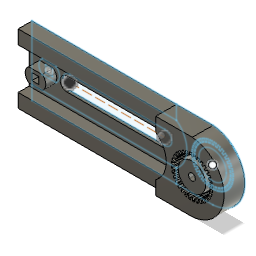
bottom slider mod v1 (Autodesk Fusion 360 design; units mm, degrees)
Autodesk Fusion 360 part; units mm, degrees
sketch "Sketch1" plane through (0, 0, 0) normal (0, 0, 1) x (1, 0, 0)
  line L0 (75, 100) -> (180, 100)
  line L1 (180, 50) -> (75, 50)
  line L2 (75, 50) -> (75, 100)
  line L3 (75, 90) -> (180, 90)
  line L4 (180, 60) -> (75, 60)
  line L5 (85, 77.5) -> (90, 77.5)
  line L6 (90, 77.5) -> (90, 72.5)
  line L7 (90, 72.5) -> (85, 72.5)
  line L8 (85, 72.5) -> (85, 77.5)
  line L9 (82.5, 80) -> (92.5, 80)
  line L10 (92.5, 70) -> (82.5, 70)
  arc A0 (92.5, 70) -> (92.5, 80) centre (88.95, 75) ccw
  arc A1 (82.5, 80) -> (82.5, 70) centre (86.5264, 75) ccw
  line L11 (102.5027, 70) -> (171.6242, 70)
  arc A2 (171.6242, 70) -> (171.6242, 80) centre (171.6242, 75) ccw
  line L12 (171.6242, 80) -> (102.5027, 80)
  arc A3 (102.5027, 80) -> (102.5027, 70) centre (102.5027, 75) ccw
  line L13 (102.5027, 75) -> (171.6242, 75) construction
  arc A4 (180, 60) -> (180, 90) centre (169.0621, 75) ccw
  circle A5 centre (206.3179, 75) radius 10
  circle A6 centre (206.3179, 75) radius 2.5
  line L14 (180, 100) -> (206.5662, 100.0787)
  line L15 (180, 50) -> (206.5662, 50)
  arc A7 (206.5662, 50) -> (206.5662, 100.0787) centre (204.5271, 75.0393) ccw
  line L16 (205.8664, 89.9932) -> (206.0662, 88.0032)
  line L17 (206.0662, 88.0032) -> (207.0662, 88.0032)
  line L18 (207.0662, 88.0032) -> (207.4096, 89.9602)
  line L19 (202.95, 89.617) -> (203.5343, 87.7043)
  line L20 (203.5343, 87.7043) -> (204.5151, 87.8993)
  line L21 (204.5151, 87.8993) -> (204.47, 89.8857)
  line L22 (200.1631, 88.6791) -> (201.1093, 86.9171)
  line L23 (201.1093, 86.9171) -> (202.0332, 87.2998)
  line L24 (202.0332, 87.2998) -> (201.6014, 89.2392)
  line L25 (197.6127, 87.2155) -> (198.8845, 85.6719)
  line L26 (198.8845, 85.6719) -> (199.7159, 86.2275)
  line L27 (199.7159, 86.2275) -> (198.9141, 88.0455)
  line L28 (195.3968, 85.2825) -> (196.9453, 84.0167)
  line L29 (196.9453, 84.0167) -> (197.6524, 84.7238)
  line L30 (197.6524, 84.7238) -> (196.5114, 86.3504)
  line L31 (193.6007, 82.9543) -> (195.3663, 82.0149)
  line L32 (195.3663, 82.0149) -> (195.9219, 82.8464)
  line L33 (195.9219, 82.8464) -> (194.4854, 84.2191)
  line L34 (192.2932, 80.3204) -> (194.2082, 79.7436)
  line L35 (194.2082, 79.7436) -> (194.5909, 80.6675)
  line L36 (194.5909, 80.6675) -> (192.9142, 81.7336)
  line L37 (191.5247, 77.4821) -> (193.5155, 77.2899)
  line L38 (193.5155, 77.2899) -> (193.7106, 78.2707)
  line L39 (193.7106, 78.2707) -> (191.8581, 78.9893)
  line L40 (191.3247, 74.5484) -> (193.3147, 74.7483)
  line L41 (193.3147, 74.7483) -> (193.3147, 75.7483)
  line L42 (193.3147, 75.7483) -> (191.3577, 76.0916)
  line L43 (191.7009, 71.6321) -> (193.6137, 72.2163)
  line L44 (193.6137, 72.2163) -> (193.4186, 73.1971)
  line L45 (193.4186, 73.1971) -> (191.4322, 73.1521)
  line L46 (192.6388, 68.8451) -> (194.4008, 69.7914)
  line L47 (194.4008, 69.7914) -> (194.0182, 70.7152)
  line L48 (194.0182, 70.7152) -> (192.0787, 70.2835)
  line L49 (194.1024, 66.2948) -> (195.646, 67.5665)
  line L50 (195.646, 67.5665) -> (195.0904, 68.398)
  line L51 (195.0904, 68.398) -> (193.2725, 67.5962)
  line L52 (196.0354, 64.0789) -> (197.3012, 65.6274)
  line L53 (197.3012, 65.6274) -> (196.5941, 66.3345)
  line L54 (196.5941, 66.3345) -> (194.9675, 65.1934)
  line L55 (198.3636, 62.2827) -> (199.303, 64.0484)
  line L56 (199.303, 64.0484) -> (198.4715, 64.604)
  line L57 (198.4715, 64.604) -> (197.0988, 63.1675)
  line L58 (200.9975, 60.9753) -> (201.5743, 62.8903)
  line L59 (201.5743, 62.8903) -> (200.6505, 63.273)
  line L60 (200.6505, 63.273) -> (199.5844, 61.5963)
  line L61 (203.8358, 60.2068) -> (204.028, 62.1975)
  line L62 (204.028, 62.1975) -> (203.0472, 62.3926)
  line L63 (203.0472, 62.3926) -> (202.3287, 60.5402)
  line L64 (206.7695, 60.0068) -> (206.5696, 61.9968)
  line L65 (206.5696, 61.9968) -> (205.5696, 61.9968)
  line L66 (205.5696, 61.9968) -> (205.2263, 60.0398)
  line L67 (209.6859, 60.383) -> (209.1016, 62.2957)
  line L68 (209.1016, 62.2957) -> (208.1208, 62.1007)
  line L69 (208.1208, 62.1007) -> (208.1659, 60.1143)
  line L70 (212.4728, 61.3209) -> (211.5266, 63.0829)
  line L71 (211.5266, 63.0829) -> (210.6027, 62.7002)
  line L72 (210.6027, 62.7002) -> (211.0344, 60.7608)
  line L73 (215.0232, 62.7845) -> (213.7514, 64.3281)
  line L74 (213.7514, 64.3281) -> (212.9199, 63.7725)
  line L75 (212.9199, 63.7725) -> (213.7217, 61.9545)
  line L76 (217.239, 64.7175) -> (215.6906, 65.9833)
  line L77 (215.6906, 65.9833) -> (214.9835, 65.2762)
  line L78 (214.9835, 65.2762) -> (216.1245, 63.6496)
  line L79 (219.0352, 67.0457) -> (217.2695, 67.9851)
  line L80 (217.2695, 67.9851) -> (216.714, 67.1536)
  line L81 (216.714, 67.1536) -> (218.1504, 65.7809)
  line L82 (220.3427, 69.6796) -> (218.4277, 70.2564)
  line L83 (218.4277, 70.2564) -> (218.045, 69.3325)
  line L84 (218.045, 69.3325) -> (219.7216, 68.2664)
  line L85 (221.1111, 72.5179) -> (219.1204, 72.7101)
  line L86 (219.1204, 72.7101) -> (218.9253, 71.7293)
  line L87 (218.9253, 71.7293) -> (220.7777, 71.0107)
  line L88 (221.3111, 75.4516) -> (219.3211, 75.2517)
  line L89 (219.3211, 75.2517) -> (219.3211, 74.2517)
  line L90 (219.3211, 74.2517) -> (221.2782, 73.9084)
  line L91 (220.9349, 78.3679) -> (219.0222, 77.7837)
  line L92 (219.0222, 77.7837) -> (219.2173, 76.8029)
  line L93 (219.2173, 76.8029) -> (221.2037, 76.8479)
  line L94 (219.997, 81.1549) -> (218.235, 80.2086)
  line L95 (218.235, 80.2086) -> (218.6177, 79.2848)
  line L96 (218.6177, 79.2848) -> (220.5571, 79.7165)
  line L97 (218.5334, 83.7052) -> (216.9899, 82.4335)
  line L98 (216.9899, 82.4335) -> (217.5454, 81.602)
  line L99 (217.5454, 81.602) -> (219.3634, 82.4038)
  line L100 (216.6004, 85.9211) -> (215.3346, 84.3726)
  line L101 (215.3346, 84.3726) -> (216.0417, 83.6655)
  line L102 (216.0417, 83.6655) -> (217.6683, 84.8066)
  line L103 (214.2722, 87.7173) -> (213.3329, 85.9516)
  line L104 (213.3329, 85.9516) -> (214.1643, 85.396)
  line L105 (214.1643, 85.396) -> (215.5371, 86.8325)
  line L106 (211.6384, 89.0247) -> (211.0615, 87.1097)
  line L107 (211.0615, 87.1097) -> (211.9854, 86.727)
  line L108 (211.9854, 86.727) -> (213.0515, 88.4037)
  line L109 (208.8001, 89.7932) -> (208.6079, 87.8025)
  line L110 (208.6079, 87.8025) -> (209.5887, 87.6074)
  line L111 (209.5887, 87.6074) -> (210.3072, 89.4598)
  arc A8 (211.6384, 89.0247) -> (210.3072, 89.4598) centre (206.3179, 75) ccw
  arc A9 (214.2722, 87.7173) -> (213.0515, 88.4037) centre (206.3179, 75) ccw
  arc A10 (216.6004, 85.9211) -> (215.5371, 86.8325) centre (206.3179, 75) ccw
  arc A11 (218.5334, 83.7052) -> (217.6683, 84.8066) centre (206.3179, 75) ccw
  arc A12 (219.997, 81.1549) -> (219.3634, 82.4038) centre (206.3179, 75) ccw
  arc A13 (220.9349, 78.3679) -> (220.5571, 79.7165) centre (206.3179, 75) ccw
  arc A14 (221.3111, 75.4516) -> (221.2037, 76.8479) centre (206.3179, 75) ccw
  arc A15 (221.1111, 72.5179) -> (221.2782, 73.9084) centre (206.3179, 75) ccw
  arc A16 (220.3427, 69.6796) -> (220.7777, 71.0107) centre (206.3179, 75) ccw
  arc A17 (219.0352, 67.0457) -> (219.7216, 68.2664) centre (206.3179, 75) ccw
  arc A18 (217.239, 64.7175) -> (218.1504, 65.7809) centre (206.3179, 75) ccw
  arc A19 (215.0232, 62.7845) -> (216.1245, 63.6496) centre (206.3179, 75) ccw
  arc A20 (212.4728, 61.3209) -> (213.7217, 61.9545) centre (206.3179, 75) ccw
  arc A21 (209.6859, 60.383) -> (211.0344, 60.7608) centre (206.3179, 75) ccw
  arc A22 (206.7695, 60.0068) -> (208.1659, 60.1143) centre (206.3179, 75) ccw
  arc A23 (203.8358, 60.2068) -> (205.2263, 60.0398) centre (206.3179, 75) ccw
  arc A24 (200.9975, 60.9753) -> (202.3287, 60.5402) centre (206.3179, 75) ccw
  arc A25 (198.3636, 62.2827) -> (199.5844, 61.5963) centre (206.3179, 75) ccw
  arc A26 (196.0354, 64.0789) -> (197.0988, 63.1675) centre (206.3179, 75) ccw
  arc A27 (194.1024, 66.2948) -> (194.9675, 65.1934) centre (206.3179, 75) ccw
  arc A28 (192.6388, 68.8451) -> (193.2725, 67.5962) centre (206.3179, 75) ccw
  arc A29 (191.7009, 71.6321) -> (192.0787, 70.2835) centre (206.3179, 75) ccw
  arc A30 (191.3247, 74.5484) -> (191.4322, 73.1521) centre (206.3179, 75) ccw
  arc A31 (191.5247, 77.4821) -> (191.3577, 76.0916) centre (206.3179, 75) ccw
  arc A32 (192.2932, 80.3204) -> (191.8581, 78.9893) centre (206.3179, 75) ccw
  arc A33 (193.6007, 82.9543) -> (192.9142, 81.7336) centre (206.3179, 75) ccw
  arc A34 (195.3968, 85.2825) -> (194.4854, 84.2191) centre (206.3179, 75) ccw
  arc A35 (197.6127, 87.2155) -> (196.5114, 86.3504) centre (206.3179, 75) ccw
  arc A36 (200.1631, 88.6791) -> (198.9141, 88.0455) centre (206.3179, 75) ccw
  arc A37 (202.95, 89.617) -> (201.6014, 89.2392) centre (206.3179, 75) ccw
  arc A38 (208.8001, 89.7932) -> (207.4096, 89.9602) centre (206.3179, 75) ccw
  arc A39 (205.8664, 89.9932) -> (204.47, 89.8857) centre (206.3179, 75) ccw
  line L112 (180, 100) -> (180, 90)
  line L113 (180, 60) -> (180, 50)
  dimension "d1" = 105
  dimension "d2" = 50
  dimension "d3" = 10
  dimension "d4" = 10
  dimension "d6" = 5
  dimension "d7" = 5
  dimension "d9" = 10
  dimension "d10" = 10
  dimension "d14" = 10
  dimension "d15" = 20
  dimension "d16" = 30
  dimension "d17" = 5
  dimension "d18" = 2
  dimension "d20" = 1
  dimension "d23" = 360
  constraint horizontal L0
  constraint vertical L112
  constraint horizontal L1
  constraint vertical L2
  constraint coincident L2 L3.start
  constraint perpendicular L2 L3
  constraint coincident L4.start L112
  constraint coincident L2 L4.end
  constraint perpendicular L2 L4
  constraint horizontal L5
  constraint vertical L6
  constraint horizontal L7
  constraint vertical L8
  constraint horizontal L9
  constraint horizontal L10
  constraint tangent L11 A2
  constraint tangent A2 L12
  constraint parallel L11 L12
  constraint tangent L12 A3
  constraint tangent L11 A3
  constraint concentric A5 A38
  constraint concentric A5 A6
  constraint coincident L16.start A38
  constraint concentric A8 A38
  constraint concentric A9 A38
  constraint concentric A10 A38
  constraint concentric A11 A38
  constraint concentric A12 A38
  constraint concentric A13 A38
  constraint concentric A14 A38
  constraint concentric A15 A38
  constraint concentric A16 A38
  constraint concentric A17 A38
  constraint concentric A18 A38
  constraint concentric A19 A38
  constraint concentric A20 A38
  constraint concentric A21 A38
  constraint concentric A22 A38
  constraint concentric A23 A38
  constraint concentric A24 A38
  constraint concentric A25 A38
  constraint concentric A26 A38
  constraint concentric A27 A38
  constraint concentric A28 A38
  constraint concentric A29 A38
  constraint concentric A30 A38
  constraint concentric A31 A38
  constraint concentric A32 A38
  constraint concentric A33 A38
  constraint concentric A34 A38
  constraint concentric A35 A38
  constraint concentric A36 A38
  constraint concentric A37 A38
  constraint concentric A38 A39
  constraint collinear L112 L113
  measures "d1" distance of L0.start L0.end
  measures "d2" distance of L0.end L1.start
  measures "d3" distance of L0 L3
  measures "d4" distance of L1 L4
  measures "d6" distance of L5.start L5.end
  measures "d7" distance of L5.end L6.end
  measures "d9" distance of L9.start L9.end
  measures "d10" distance of L9.start L10.end
  measures "d14" diameter of A2
  measures "d15" diameter of A5
  measures "d16" diameter of A38
  measures "d17" diameter of A6
  measures "d18" distance of L16.start L16.end
  measures "d20" distance of L16.end L17.end
extrude "Extrude1" add sketch "Sketch1" along normal blind 10 contours L0 L2 L3 L112 | L1 L2 L4 L113 | L9 L10 A0 A1 makes body 1 at (110, 100, 3.3333) makes body 2 at (93.4039, 79.2148, 6.6667) makes body 3 at (145, 53.3333, 0)
extrude "Extrude2" add sketch "Sketch1" along normal blind 2 contours L2 L3 L4 A4 bodies 1 2 3
extrude "Extrude3" add sketch "Sketch1" along normal blind 15 contours A4 L14 L15 A7 L112 L113 | A5 bodies 1 makes body 4 at (216.2682, 74.0043, 10)
extrude "Extrude4" add sketch "Sketch1" along normal blind 2 contours L16 L17 L18 L19 L20 L21 L22 L23 L24 L25 L26 L27 L28 L29 L30 L31 L32 L33 L34 L35 L36 L37 L38 L39 L40 L41 L42 L43 L44 L45 L46 L47 L48 L49 L50 L51 L52 L53 L54 L55 L56 L57 L58 L59 L60 L61 L62 L63 L64 L65 L66 L67 L68 L69 L70 L71 L72 L73 L74 L75 L76 L77 L78 L79 L80 L81 L82 L83 L84 L85 L86 L87 L88 L89 L90 L91 L92 L93 L94 L95 L96 L97 L98 L99 L100 L101 L102 L103 L104 L105 L106 L107 L108 L109 L110 L111 A8 A9 A10 A11 A12 A13 A14 A15 A16 A17 A18 A19 A20 A21 A22 A23 A24 A25 A26 A27 A28 A29 A30 A31 A32 A33 A34 A35 A36 A37 A38 A39 bodies 1 4
